Autodesk Fusion 360 part; units mm, degrees
(part 2 of 3)
  arc A65 (20.2, 68) -> (20, 67.8) centre (20.2, 67.8) ccw
  line L946 (26, 62.4) -> (26.5, 62.4)
  line L947 (20, 62.2) -> (20, 63.55)
  line L948 (26, 63.1) -> (26, 62.4)
  arc A66 (37.0205, 29.8133) -> (36.6712, 29.464) centre (37.0205, 29.464) ccw
  line L949 (37.2921, 29.6968) -> (38.0682, 29.0371)
  line L950 (25.75, 68) -> (25.8, 68)
  arc A67 (37.2921, 26.9628) -> (36.6713, 26.9628) centre (36.9817, 26.9628) ccw
  line L951 (37.7578, 23.9571) -> (37.7578, 24.7333)
  line L952 (44.4112, 30.9247) -> (43.7903, 30.9247)
  line L953 (38.0682, 31.3231) -> (38.0682, 32.0993)
  line L954 (44.7993, 33.1153) -> (43.4023, 33.1153)
  line L955 (19.5, 67.6) -> (19.5, 66.9)
  line L956 (36.6713, 31.7112) -> (38.0682, 31.7112)
  arc A68 (43.7903, 31.7008) -> (43.7903, 30.9246) centre (43.7903, 31.3127) ccw
  arc A69 (38.0683, 26.8852) -> (37.2921, 26.8852) centre (37.6802, 26.8852) ccw
  line L957 (38.0682, 26.4971) -> (38.0682, 26.8852)
  arc A70 (26, 67.8) -> (25.8, 68) centre (25.8, 67.8) ccw
  line L958 (44.7993, 32.3391) -> (43.4023, 32.3391)
  line L959 (37.2921, 26.9628) -> (37.2921, 26.6524)
  line L960 (36.6713, 24.2676) -> (37.7578, 23.9571)
  line L961 (38.0682, 29.0371) -> (38.0682, 29.8133)
  arc A71 (36.6712, 29.464) -> (36.9817, 29.0371) centre (37.1199, 29.464) ccw
  line L962 (37.4474, 24.5004) -> (38.0682, 24.5004)
  line L963 (43.4023, 32.3391) -> (44.7993, 33.1153)
  line L964 (20, 63.1) -> (19.5, 63.1)
  line L965 (19.5, 66.9) -> (20, 66.9)
  line L966 (36.6713, 26.4971) -> (36.6713, 26.9628)
  line L967 (26.5, 63.1) -> (26, 63.1)
  line L968 (25.8, 62) -> (25.4, 62)
  line L969 (40.8, 53.3) -> (39.2, 53.3)
  line L970 (36.7, 15.6) -> (38.3, 15.6)
  arc A72 (44.4112, 30.9246) -> (44.4112, 31.7008) centre (44.4112, 31.3127) ccw
  line L971 (39.2, 12) -> (40.8, 12)
  line L972 (43.3, 53.3) -> (41.7, 53.3)
  line L973 (39.2, 15.6) -> (40.8, 15.6)
  line L974 (41.7, 15.6) -> (43.3, 15.6)
  line L975 (38.3, 53.3) -> (36.7, 53.3)
  line L976 (36.9817, 31.3231) -> (36.6713, 31.7112)
  line L977 (41.7, 12) -> (43.3, 12)
  arc A73 (37.2921, 29.6968) -> (37.0205, 29.8132) centre (37.0205, 29.4381) ccw
  line L978 (43.7903, 31.7008) -> (44.4112, 31.7008)
  line L979 (43.3, 49.7) -> (41.7, 49.7)
  line L980 (36.7, 12) -> (38.3, 12)
  line L981 (38.3, 49.7) -> (36.7, 49.7)
  line L982 (40.8, 49.7) -> (39.2, 49.7)
  line L983 (14.5813, 71.8525) -> (14.5813, 70.8525)
  circle A74 centre (15.0813, 71.8525) radius 0.5
  line L984 (15.5813, 70.8525) -> (15.5813, 71.8525)
  line L985 (14.5813, 57.0525) -> (15.5813, 57.0525)
  line L986 (14.5813, 70.8525) -> (15.5813, 70.8525)
  line L987 (15.5813, 71.8525) -> (14.5813, 71.8525)
  line L988 (15.5813, 57.0525) -> (15.5813, 58.0525)
  circle A75 centre (15.0813, 57.0525) radius 0.5
  line L989 (24.714, 14.816) -> (24.714, 15.324)
  line L990 (33.401, 50.419) -> (33.401, 49.911)
  line L991 (24.206, 15.324) -> (24.206, 14.816)
  line L992 (26.746, 14.816) -> (27.254, 14.816)
  line L993 (33.401, 52.959) -> (33.401, 52.451)
  line L994 (33.909, 52.959) -> (33.401, 52.959)
  line L995 (24.714, 15.324) -> (24.206, 15.324)
  line L996 (27.254, 15.324) -> (26.746, 15.324)
  line L997 (14.5813, 58.0525) -> (14.5813, 57.0525)
  line L998 (15.5813, 58.0525) -> (14.5813, 58.0525)
  line L999 (33.909, 50.419) -> (33.401, 50.419)
  line L1000 (33.909, 52.451) -> (33.909, 52.959)
  line L1001 (33.909, 49.911) -> (33.909, 50.419)
  line L1002 (33.401, 49.911) -> (33.909, 49.911)
  line L1003 (33.401, 52.451) -> (33.909, 52.451)
  line L1004 (24.206, 14.816) -> (24.714, 14.816)
  line L1005 (27.254, 14.816) -> (27.254, 15.324)
  line L1006 (24.714, 12.276) -> (24.714, 12.784)
  line L1007 (24.714, 12.784) -> (24.206, 12.784)
  line L1008 (24.206, 12.784) -> (24.206, 12.276)
  line L1009 (24.206, 12.276) -> (24.714, 12.276)
sketch "PET_Diag_Clip" plane through (0, 0, 0) normal (0, 0, 1) x (1, 0, 0) in component "PCB"
  line L0 (0, 0) -> (47, 0)
  line L1 (0, 77) -> (0, 0)
  line L2 (47, 0) -> (47, 77)
  line L3 (47, 77) -> (0, 77)
  line L4 (7.366, 50.434) -> (7.366, 49.926)
  line L5 (7.874, 50.434) -> (7.366, 50.434)
  line L6 (7.874, 47.386) -> (7.874, 47.894)
  line L7 (4.826, 44.846) -> (5.334, 44.846)
  line L8 (7.874, 57.546) -> (7.874, 58.054)
  line L9 (4.826, 55.514) -> (4.826, 55.006)
  line L10 (7.366, 57.546) -> (7.874, 57.546)
  line L11 (4.826, 45.354) -> (4.826, 44.846)
  line L12 (7.874, 58.054) -> (7.366, 58.054)
  line L13 (7.366, 47.894) -> (7.366, 47.386)
  line L14 (4.826, 50.434) -> (4.826, 49.926)
  line L15 (7.366, 52.466) -> (7.874, 52.466)
  line L16 (7.874, 45.354) -> (7.366, 45.354)
  line L17 (7.874, 44.846) -> (7.874, 45.354)
  line L18 (7.874, 55.006) -> (7.874, 55.514)
  line L19 (7.366, 52.974) -> (7.366, 52.466)
  line L20 (5.334, 47.894) -> (4.826, 47.894)
  line L21 (7.366, 49.926) -> (7.874, 49.926)
  line L22 (5.334, 57.546) -> (5.334, 58.054)
  line L23 (5.334, 58.054) -> (4.826, 58.054)
  line L24 (7.874, 42.306) -> (7.874, 42.814)
  line L25 (5.334, 49.926) -> (5.334, 50.434)
  line L26 (7.366, 42.306) -> (7.874, 42.306)
  line L27 (7.366, 58.054) -> (7.366, 57.546)
  line L28 (4.826, 52.466) -> (5.334, 52.466)
  line L29 (7.366, 44.846) -> (7.874, 44.846)
  line L30 (4.826, 57.546) -> (5.334, 57.546)
  line L31 (5.334, 52.466) -> (5.334, 52.974)
  line L32 (5.334, 50.434) -> (4.826, 50.434)
  line L33 (7.874, 60.086) -> (7.874, 60.594)
  line L34 (5.334, 47.386) -> (5.334, 47.894)
  line L35 (5.334, 45.354) -> (4.826, 45.354)
  line L36 (5.334, 55.006) -> (5.334, 55.514)
  line L37 (4.826, 47.894) -> (4.826, 47.386)
  line L38 (7.366, 47.386) -> (7.874, 47.386)
  line L39 (7.366, 55.006) -> (7.874, 55.006)
  line L40 (7.874, 60.594) -> (7.366, 60.594)
  line L41 (4.826, 47.386) -> (5.334, 47.386)
  line L42 (4.826, 55.006) -> (5.334, 55.006)
  line L43 (7.366, 55.514) -> (7.366, 55.006)
  line L44 (4.826, 52.974) -> (4.826, 52.466)
  line L45 (7.874, 52.466) -> (7.874, 52.974)
  line L46 (7.874, 49.926) -> (7.874, 50.434)
  line L47 (5.334, 44.846) -> (5.334, 45.354)
  line L48 (7.366, 42.814) -> (7.366, 42.306)
  line L49 (4.826, 58.054) -> (4.826, 57.546)
  line L50 (5.334, 55.514) -> (4.826, 55.514)
  line L51 (7.874, 52.974) -> (7.366, 52.974)
  line L52 (5.334, 52.974) -> (4.826, 52.974)
  line L53 (7.874, 47.894) -> (7.366, 47.894)
  line L54 (7.874, 55.514) -> (7.366, 55.514)
  line L55 (4.826, 49.926) -> (5.334, 49.926)
  line L56 (4.826, 60.594) -> (4.826, 60.086)
  line L57 (7.366, 45.354) -> (7.366, 44.846)
  line L58 (4.826, 32.654) -> (4.826, 32.146)
  line L59 (7.874, 34.686) -> (7.874, 35.194)
  line L60 (7.366, 34.686) -> (7.874, 34.686)
  line L61 (5.334, 42.814) -> (4.826, 42.814)
  line L62 (4.826, 37.734) -> (4.826, 37.226)
  line L63 (7.366, 39.766) -> (7.874, 39.766)
  line L64 (4.826, 30.114) -> (4.826, 29.606)
  line L65 (7.366, 62.626) -> (7.874, 62.626)
  line L66 (7.366, 60.086) -> (7.874, 60.086)
  line L67 (7.874, 39.766) -> (7.874, 40.274)
  line L68 (7.874, 37.226) -> (7.874, 37.734)
  line L69 (7.874, 40.274) -> (7.366, 40.274)
  line L70 (7.366, 37.734) -> (7.366, 37.226)
  line L71 (7.366, 27.066) -> (7.874, 27.066)
  line L72 (7.874, 37.734) -> (7.366, 37.734)
  line L73 (4.826, 35.194) -> (4.826, 34.686)
  line L74 (5.334, 63.134) -> (4.826, 63.134)
  line L75 (5.334, 35.194) -> (4.826, 35.194)
  line L76 (5.334, 60.086) -> (5.334, 60.594)
  line L77 (5.334, 60.594) -> (4.826, 60.594)
  line L78 (7.874, 27.066) -> (7.874, 27.574)
  line L79 (4.826, 29.606) -> (5.334, 29.606)
  line L80 (4.826, 63.134) -> (4.826, 62.626)
  line L81 (7.874, 27.574) -> (7.366, 27.574)
  line L82 (5.334, 32.654) -> (4.826, 32.654)
  line L83 (4.826, 39.766) -> (5.334, 39.766)
  line L84 (7.366, 30.114) -> (7.366, 29.606)
  line L85 (4.826, 27.574) -> (4.826, 27.066)
  line L86 (7.874, 63.134) -> (7.366, 63.134)
  line L87 (7.366, 60.594) -> (7.366, 60.086)
  line L88 (4.826, 62.626) -> (5.334, 62.626)
  line L89 (5.334, 62.626) -> (5.334, 63.134)
  line L90 (5.334, 34.686) -> (5.334, 35.194)
  line L91 (5.334, 32.146) -> (5.334, 32.654)
  line L92 (4.826, 27.066) -> (5.334, 27.066)
  line L93 (7.366, 29.606) -> (7.874, 29.606)
  line L94 (4.826, 60.086) -> (5.334, 60.086)
  line L95 (7.366, 32.146) -> (7.874, 32.146)
  line L96 (7.366, 63.134) -> (7.366, 62.626)
  line L97 (4.826, 34.686) -> (5.334, 34.686)
  line L98 (7.874, 42.814) -> (7.366, 42.814)
  line L99 (7.366, 35.194) -> (7.366, 34.686)
  line L100 (7.366, 40.274) -> (7.366, 39.766)
  line L101 (7.366, 37.226) -> (7.874, 37.226)
  line L102 (7.874, 62.626) -> (7.874, 63.134)
  line L103 (7.874, 35.194) -> (7.366, 35.194)
  line L104 (5.334, 39.766) -> (5.334, 40.274)
  line L105 (7.874, 30.114) -> (7.366, 30.114)
  line L106 (5.334, 19.954) -> (4.826, 19.954)
  line L107 (7.366, 19.446) -> (7.874, 19.446)
  line L108 (7.366, 14.874) -> (7.366, 14.366)
  line L109 (4.826, 40.274) -> (4.826, 39.766)
  line L110 (4.826, 32.146) -> (5.334, 32.146)
  line L111 (4.826, 25.034) -> (4.826, 24.526)
  line L112 (7.874, 24.526) -> (7.874, 25.034)
  line L113 (4.826, 24.526) -> (5.334, 24.526)
  line L114 (7.366, 27.574) -> (7.366, 27.066)
  line L115 (5.334, 29.606) -> (5.334, 30.114)
  line L116 (4.826, 42.306) -> (5.334, 42.306)
  line L117 (7.366, 25.034) -> (7.366, 24.526)
  line L118 (5.334, 40.274) -> (4.826, 40.274)
  line L119 (5.334, 37.226) -> (5.334, 37.734)
  line L120 (7.366, 14.366) -> (7.874, 14.366)
  line L121 (7.874, 29.606) -> (7.874, 30.114)
  line L122 (7.366, 21.986) -> (7.874, 21.986)
  line L123 (5.334, 37.734) -> (4.826, 37.734)
  line L124 (7.366, 32.654) -> (7.366, 32.146)
  line L125 (4.826, 42.814) -> (4.826, 42.306)
  line L126 (7.874, 16.906) -> (7.874, 17.414)
  line L127 (7.366, 17.414) -> (7.366, 16.906)
  line L128 (5.334, 22.494) -> (4.826, 22.494)
  line L129 (5.334, 30.114) -> (4.826, 30.114)
  line L130 (5.334, 14.874) -> (4.826, 14.874)
  line L131 (7.874, 22.494) -> (7.366, 22.494)
  line L132 (4.826, 37.226) -> (5.334, 37.226)
  line L133 (4.826, 22.494) -> (4.826, 21.986)
  line L134 (7.874, 32.654) -> (7.366, 32.654)
  line L135 (7.874, 32.146) -> (7.874, 32.654)
  line L136 (5.334, 42.306) -> (5.334, 42.814)
  line L137 (7.366, 24.526) -> (7.874, 24.526)
  line L138 (5.334, 24.526) -> (5.334, 25.034)
  line L139 (5.334, 27.066) -> (5.334, 27.574)
  line L140 (5.334, 17.414) -> (4.826, 17.414)
  line L141 (7.366, 16.906) -> (7.874, 16.906)
  line L142 (7.874, 25.034) -> (7.366, 25.034)
  line L143 (4.826, 17.414) -> (4.826, 16.906)
  line L144 (5.334, 14.366) -> (5.334, 14.874)
  line L145 (5.334, 21.986) -> (5.334, 22.494)
  line L146 (5.334, 27.574) -> (4.826, 27.574)
  line L147 (7.874, 14.366) -> (7.874, 14.874)
  line L148 (4.826, 21.986) -> (5.334, 21.986)
  line L149 (7.874, 19.954) -> (7.366, 19.954)
  line L150 (5.334, 19.446) -> (5.334, 19.954)
  line L151 (7.874, 21.986) -> (7.874, 22.494)
  line L152 (7.874, 14.874) -> (7.366, 14.874)
  line L153 (7.366, 22.494) -> (7.366, 21.986)
  line L154 (4.826, 14.874) -> (4.826, 14.366)
  line L155 (5.334, 25.034) -> (4.826, 25.034)
  line L156 (4.826, 16.906) -> (5.334, 16.906)
  line L157 (7.874, 17.414) -> (7.366, 17.414)
  line L158 (4.826, 19.446) -> (5.334, 19.446)
  line L159 (5.334, 16.906) -> (5.334, 17.414)
  line L160 (4.826, 14.366) -> (5.334, 14.366)
  line L161 (7.874, 19.446) -> (7.874, 19.954)
  line L162 (7.366, 19.954) -> (7.366, 19.446)
  line L163 (4.826, 19.954) -> (4.826, 19.446)
  line L164 (17.8813, 69.2525) -> (17.8813, 59.6525)
  line L165 (17.8813, 59.6525) -> (12.2813, 59.6525)
  line L166 (12.2813, 59.6525) -> (12.2813, 69.2525)
  line L167 (12.2813, 69.2525) -> (17.8813, 69.2525)
  circle A0 centre (5, 5) radius 3.1789
  circle A1 centre (5, 5) radius 1.7463
  circle A2 centre (42, 5) radius 3.1789
  circle A3 centre (42, 5) radius 1.7463
  circle A4 centre (42, 72) radius 3.1789
  circle A5 centre (42, 72) radius 1.7463
  circle A6 centre (5, 72) radius 3.1789
  circle A7 centre (5, 72) radius 1.7463
  line L168 (23.3362, 18.542) -> (28.6703, 18.542)
  arc A8 (23.3363, 18.542) -> (20.7963, 18.542) centre (22.0663, 18.542) ccw
  line L169 (28.6703, 53.848) -> (15.4623, 53.848)
  line L170 (15.4623, 18.542) -> (20.7963, 18.542)
  line L171 (15.4623, 18.542) -> (15.4623, 53.848)
  line L172 (28.6703, 18.542) -> (28.6703, 53.848)
  line L173 (35.687, 9.398) -> (16.383, 9.398)
  line L174 (16.383, 3.302) -> (35.687, 3.302)
  line L175 (35.687, 9.398) -> (35.687, 3.302)
  line L176 (16.383, 9.398) -> (16.383, 7.366)
  line L177 (16.383, 3.302) -> (16.383, 5.334)
  arc A9 (16.383, 5.334) -> (16.383, 7.366) centre (16.383, 6.35) ccw
  line L178 (10.9538, 67.96) -> (10.9538, 9.54)
  line L179 (10.9538, 9.54) -> (9.525, 9.54)
  line L180 (9.525, 9.54) -> (8.0963, 9.54)
  line L181 (8.0963, 9.54) -> (1.7462, 9.54)
  line L182 (1.7462, 9.54) -> (1.7462, 36.6862)
  line L183 (1.7462, 36.6862) -> (1.7462, 40.8138)
  line L184 (1.7462, 40.8138) -> (1.7462, 62.0863)
  line L185 (1.7462, 62.0863) -> (1.7462, 62.4038)
  line L186 (1.7462, 62.4038) -> (1.7462, 62.5625)
  line L187 (1.7462, 62.5625) -> (1.7462, 62.7213)
  line L188 (1.7462, 62.7213) -> (1.7462, 62.88)
  line L189 (1.7462, 62.88) -> (1.7462, 63.0388)
  line L190 (1.7462, 63.1975) -> (1.7462, 63.3563)
  line L191 (1.7462, 63.3563) -> (1.7462, 63.515)
  line L192 (1.7462, 63.515) -> (1.7462, 63.6738)
  line L193 (1.7462, 63.6738) -> (1.7462, 67.96)
  line L194 (1.7462, 67.96) -> (8.0963, 67.96)
  line L195 (8.0963, 67.96) -> (9.525, 67.96)
  line L196 (9.525, 67.96) -> (10.9538, 67.96)
  line L197 (9.6838, 66.69) -> (9.6838, 10.81)
  line L198 (9.6838, 10.81) -> (9.525, 10.81)
  line L199 (9.525, 10.81) -> (8.0963, 10.81)
  line L200 (8.0963, 10.81) -> (3.0162, 10.81)
  line L201 (3.0162, 10.81) -> (3.0162, 36.6862)
  line L202 (3.0162, 36.6862) -> (3.0162, 40.8138)
  line L203 (3.0162, 40.8138) -> (3.0162, 66.69)
  line L204 (3.0162, 66.69) -> (8.0963, 66.69)
  line L205 (8.0963, 66.69) -> (9.525, 66.69)
  line L206 (9.525, 66.69) -> (9.6838, 66.69)
  line L207 (3.0162, 40.8138) -> (2.54, 40.8138)
  line L208 (2.54, 40.8138) -> (1.7462, 40.8138)
  line L209 (3.0162, 36.6862) -> (2.54, 36.6862)
  line L210 (2.54, 36.6862) -> (1.7462, 36.6862)
  line L211 (9.525, 10.81) -> (9.525, 10.3337)
  line L212 (9.525, 10.3337) -> (9.525, 9.54)
  line L213 (9.525, 66.69) -> (9.525, 67.1663)
  line L214 (9.525, 67.1663) -> (9.525, 67.96)
  line L215 (8.0963, 66.69) -> (8.0963, 67.1663)
  line L216 (8.0963, 67.1663) -> (8.0963, 67.96)
  line L217 (8.0963, 10.81) -> (8.0963, 10.3337)
  line L218 (8.0963, 10.3337) -> (8.0963, 9.54)
  line L219 (10.16, 67.1663) -> (10.16, 10.3337)
  line L220 (2.54, 36.6862) -> (2.54, 10.3337)
  line L221 (8.0963, 10.3337) -> (2.54, 10.3337)
  line L222 (10.16, 67.1663) -> (9.525, 67.1663)
  line L223 (8.0963, 67.1663) -> (2.54, 67.1663)
  line L224 (2.54, 40.8138) -> (2.54, 62.88)
  line L225 (2.54, 62.88) -> (2.54, 67.1663)
  line L226 (9.525, 10.3337) -> (10.16, 10.3337)
  line L227 (3.0162, 10.81) -> (2.54, 10.3337)
  line L228 (9.6838, 10.81) -> (10.16, 10.3337)
  line L229 (10.16, 67.1663) -> (9.6838, 66.69)
  line L230 (2.54, 67.1663) -> (3.0162, 66.69)
  arc A10 (10.9538, 65.42) -> (10.9538, 66.69) centre (10.9538, 66.055) ccw
  arc A11 (10.9538, 10.81) -> (10.9538, 12.08) centre (10.9538, 11.445) ccw
  arc A12 (10.9538, 38.2738) -> (10.9538, 39.385) centre (10.9538, 38.8294) ccw
  line L231 (2.54, 62.88) -> (1.7462, 63.6738)
  line L232 (2.54, 62.88) -> (2.5399, 62.88)
  line L233 (2.5399, 62.88) -> (2.3812, 62.7213)
  line L234 (2.3812, 62.7213) -> (2.0637, 62.4038)
  line L235 (2.0637, 62.4038) -> (1.7462, 62.0863)
  line L236 (2.3812, 62.88) -> (1.7462, 63.515)
  line L237 (1.7462, 63.3563) -> (2.3812, 62.7213)
  line L238 (2.2225, 62.7213) -> (2.2224, 62.7213)
  line L239 (2.2224, 62.7213) -> (1.7462, 63.1975)
  line L240 (1.7462, 63.1975) -> (1.7462, 63.0388)
  line L241 (1.7462, 63.0388) -> (2.2225, 62.5625)
  line L242 (1.7462, 62.88) -> (2.0637, 62.5625)
  line L243 (1.7462, 62.7213) -> (2.0637, 62.4038)
  line L244 (1.7462, 62.5625) -> (1.7463, 62.5625)
  line L245 (1.7463, 62.5625) -> (1.905, 62.4038)
  line L246 (1.7462, 62.4038) -> (1.905, 62.245)
  arc A13 (38.5, 55.7) -> (41.5, 55.7) centre (40, 56.5) ccw
  arc A14 (41.5, 57.3) -> (38.5, 57.3) centre (40, 56.5) ccw
  arc A15 (38.5, 55.7) -> (41.5, 55.7) centre (40, 56.5) ccw
  arc A16 (41.5, 57.3) -> (38.5, 57.3) centre (40, 56.5) ccw
  line L247 (20.25, 68) -> (25.75, 68)
  line L248 (26, 66.45) -> (26, 63.6)
  line L249 (25.4, 62) -> (20.25, 62)
  line L250 (20, 63.55) -> (20, 66.45)
  arc A17 (20.55, 62.45) -> (20.5, 63.2) centre (20.8502, 62.8467) ccw
  arc A18 (20.55, 66.75) -> (20.5, 67.5) centre (20.8502, 67.1467) ccw
  arc A19 (25.45, 67.55) -> (25.5, 66.8) centre (25.1498, 67.1533) ccw
  arc A20 (25.45, 63.25) -> (25.45, 62.45) centre (25.15, 62.85) ccw
  circle A21 centre (23, 65) radius 1.75
  circle A22 centre (23, 65) radius 1.4
  line L251 (35.8458, 33.9408) -> (35.8458, 22.2568)
  line L252 (45.7518, 22.2568) -> (45.7518, 33.9408)
  line L253 (45.7518, 33.9408) -> (42.4498, 33.9408)
  line L254 (39.1478, 33.9408) -> (39.1478, 33.4327)
  line L255 (39.1478, 33.4327) -> (42.4498, 33.4327)
  line L256 (42.4498, 33.4327) -> (42.4498, 33.9408)
  line L257 (39.1478, 33.9408) -> (35.8458, 33.9408)
  line L258 (42.4498, 33.9408) -> (39.1478, 33.9408)
  line L259 (35.8458, 22.2568) -> (39.1478, 22.2568)
  line L260 (42.4498, 22.2568) -> (42.4498, 22.7647)
  line L261 (42.4498, 22.7647) -> (39.1478, 22.7647)
  line L262 (39.1478, 22.7647) -> (39.1478, 22.2568)
  line L263 (42.4498, 22.2568) -> (45.7518, 22.2568)
  line L264 (39.1478, 22.2568) -> (42.4498, 22.2568)
  line L265 (42.7037, 25.0508) -> (38.8938, 25.0508)
  line L266 (42.7037, 25.0508) -> (42.7037, 23.5267)
  line L267 (38.8938, 23.5267) -> (42.7037, 23.5267)
  line L268 (38.8938, 23.5267) -> (38.8938, 25.0508)
  line L269 (40.7988, 24.7968) -> (39.1478, 24.7968)
  line L270 (40.7988, 23.7808) -> (39.1478, 23.7808)
  line L271 (42.7037, 27.5907) -> (38.8938, 27.5907)
  line L272 (42.7037, 27.5907) -> (42.7037, 26.0668)
  line L273 (38.8938, 26.0668) -> (42.7037, 26.0668)
  line L274 (38.8938, 26.0668) -> (38.8938, 27.5907)
  line L275 (40.7988, 27.3368) -> (39.1478, 27.3368)
  line L276 (40.7988, 26.3208) -> (39.1478, 26.3208)
  line L277 (42.7037, 30.1308) -> (38.8938, 30.1308)
  line L278 (42.7037, 30.1308) -> (42.7037, 28.6068)
  line L279 (38.8938, 28.6068) -> (42.7037, 28.6068)
  line L280 (38.8938, 28.6068) -> (38.8938, 30.1308)
  line L281 (40.7988, 29.8768) -> (39.1478, 29.8768)
  line L282 (40.7988, 28.8608) -> (39.1478, 28.8608)
  line L283 (42.7037, 32.6707) -> (38.8938, 32.6707)
  line L284 (42.7037, 32.6707) -> (42.7037, 31.1468)
  line L285 (38.8938, 31.1468) -> (42.7037, 31.1468)
  line L286 (38.8938, 31.1468) -> (38.8938, 32.6707)
  line L287 (40.7988, 32.4168) -> (39.1478, 32.4168)
  line L288 (40.7988, 31.4008) -> (39.1478, 31.4008)
  line L289 (35.5, 15.6) -> (35.5, 12)
  line L290 (35.5, 12) -> (36.7, 12)
  line L291 (35.5, 15.6) -> (36.7, 15.6)
  line L292 (44.6, 12) -> (44.6, 15.6)
  line L293 (44.6, 15.6) -> (43.3, 15.6)
  line L294 (44.6, 12) -> (43.3, 12)
  line L295 (38.3, 15.6) -> (39.2, 15.6)
  line L296 (40.8, 15.6) -> (41.7, 15.6)
  line L297 (38.3, 12) -> (39.2, 12)
  line L298 (40.8, 12) -> (41.7, 12)
  line L299 (38.3, 14.5) -> (38.3, 13.1)
  line L300 (38.3, 13.1) -> (41.7, 13.1)
  line L301 (41.7, 13.1) -> (41.7, 14.5)
  line L302 (41.7, 14.5) -> (38.3, 14.5)
  line L303 (31.35, 77) -> (23.5, 77)
  line L304 (23.5, 77) -> (15.65, 77)
  line L305 (31.35, 77) -> (31.35, 83.5)
  line L306 (15.65, 77) -> (15.65, 83.5)
  line L307 (35.15, 83.9) -> (23.85, 83.9)
  line L308 (23.85, 83.9) -> (18.85, 83.9)
  line L309 (18.85, 83.9) -> (11.85, 83.9)
  line L310 (35.15, 83.5) -> (11.85, 83.5)
  line L311 (11.85, 83.9) -> (11.85, 83.5)
  line L312 (35.15, 83.9) -> (35.15, 83.5)
  line L313 (18.85, 83.9) -> (18.85, 88.4)
  line L314 (21.35, 88.9) -> (20.85, 88.4)
  line L315 (20.85, 88.4) -> (20.35, 88.9)
  line L316 (20.35, 88.9) -> (19.85, 88.4)
  line L317 (19.85, 88.4) -> (19.35, 88.9)
  line L318 (21.35, 88.9) -> (21.85, 88.4)
  line L319 (21.85, 88.4) -> (22.35, 88.9)
  line L320 (22.35, 88.9) -> (22.85, 88.4)
  line L321 (22.85, 88.4) -> (23.35, 88.9)
  line L322 (19.35, 88.9) -> (18.85, 88.4)
  line L323 (23.35, 88.9) -> (23.85, 88.4)
  line L324 (23.85, 88.4) -> (23.85, 83.9)
  line L325 (33, 86) -> (33, 84.5)
  line L326 (33, 83.5) -> (33, 82)
  line L327 (14, 86) -> (14, 84.5)
  line L328 (14, 83.5) -> (14, 82)
  line L329 (12.2813, 61.4525) -> (12.2813, 60.4525)
  line L330 (17.8813, 60.4525) -> (17.8813, 61.4525)
  line L331 (17.8813, 61.4525) -> (12.2813, 61.4525)
  line L332 (12.2813, 60.4525) -> (17.8813, 60.4525)
  line L333 (15.5813, 58.0525) -> (15.5813, 59.6525)
  line L334 (15.5813, 70.8525) -> (14.5813, 70.8525)
  line L335 (14.5813, 58.0525) -> (15.5813, 58.0525)
  line L336 (15.5813, 59.6525) -> (14.5813, 59.6525)
  line L337 (14.5813, 59.6525) -> (14.5813, 58.0525)
  line L338 (14.5813, 69.2525) -> (15.5813, 69.2525)
  line L339 (15.5813, 69.2525) -> (15.5813, 70.8525)
  line L340 (14.5813, 70.8525) -> (14.5813, 69.2525)
  line L341 (40.1638, 29.8768) -> (39.7828, 29.8768)
  line L342 (40.4178, 26.3208) -> (40.7988, 26.3208)
  line L343 (40.1638, 27.3368) -> (39.7828, 27.3368)
  line L344 (39.1478, 24.7968) -> (39.1478, 23.7808)
  line L345 (40.1638, 31.4008) -> (40.1638, 32.4168)
  line L346 (39.1478, 32.4168) -> (39.1478, 31.4008)
  line L347 (39.7828, 29.8768) -> (39.7828, 28.8608)
  line L348 (39.7828, 24.7968) -> (39.7828, 23.7808)
  line L349 (39.5288, 24.7968) -> (39.1478, 24.7968)
  line L350 (40.4178, 28.8608) -> (40.7988, 28.8608)
  line L351 (40.4178, 31.4008) -> (40.7988, 31.4008)
  line L352 (40.7988, 26.3208) -> (40.7988, 27.3368)
  line L353 (40.1638, 24.7968) -> (39.7828, 24.7968)
  line L354 (40.4178, 27.3368) -> (40.4178, 26.3208)
  line L355 (40.1638, 23.7808) -> (40.1638, 24.7968)
  line L356 (39.7828, 27.3368) -> (39.7828, 26.3208)
  line L357 (39.5288, 26.3208) -> (39.5288, 27.3368)
  line L358 (39.1478, 26.3208) -> (39.5288, 26.3208)
  line L359 (40.7988, 27.3368) -> (40.4178, 27.3368)
  line L360 (40.1638, 26.3208) -> (40.1638, 27.3368)
  line L361 (40.7988, 24.7968) -> (40.4178, 24.7968)
  line L362 (40.7988, 28.8608) -> (40.7988, 29.8768)
  line L363 (39.7828, 26.3208) -> (40.1638, 26.3208)
  line L364 (40.7988, 29.8768) -> (40.4178, 29.8768)
  line L365 (39.1478, 23.7808) -> (39.5288, 23.7808)
  line L366 (39.5288, 27.3368) -> (39.1478, 27.3368)
  line L367 (40.4178, 24.7968) -> (40.4178, 23.7808)
  line L368 (40.1638, 28.8608) -> (40.1638, 29.8768)
  line L369 (39.1478, 28.8608) -> (39.5288, 28.8608)
  line L370 (39.1478, 27.3368) -> (39.1478, 26.3208)
  line L371 (39.7828, 31.4008) -> (40.1638, 31.4008)
  line L372 (39.5288, 28.8608) -> (39.5288, 29.8768)
  line L373 (39.5288, 32.4168) -> (39.1478, 32.4168)
  line L374 (39.7828, 28.8608) -> (40.1638, 28.8608)
  line L375 (40.4178, 29.8768) -> (40.4178, 28.8608)
  line L376 (40.7988, 32.4168) -> (40.4178, 32.4168)
  line L377 (39.1478, 31.4008) -> (39.5288, 31.4008)
  line L378 (39.5288, 31.4008) -> (39.5288, 32.4168)
  line L379 (39.1478, 29.8768) -> (39.1478, 28.8608)
  line L380 (39.5288, 29.8768) -> (39.1478, 29.8768)
  line L381 (40.7988, 31.4008) -> (40.7988, 32.4168)
  line L382 (40.1638, 32.4168) -> (39.7828, 32.4168)
  line L383 (40.7988, 23.7808) -> (40.7988, 24.7968)
  line L384 (39.5288, 23.7808) -> (39.5288, 24.7968)
  line L385 (39.7828, 23.7808) -> (40.1638, 23.7808)
  line L386 (40.4178, 32.4168) -> (40.4178, 31.4008)
  line L387 (39.7828, 32.4168) -> (39.7828, 31.4008)
  line L388 (40.4178, 23.7808) -> (40.7988, 23.7808)
  line L389 (40.3, 14.5) -> (40.3, 13.1)
  line L390 (41.7, 14.5) -> (40.3, 14.5)
  line L391 (40.3, 13.1) -> (41.7, 13.1)
  line L392 (41.7, 13.1) -> (41.7, 14.5)
  line L393 (19.5, 67.6) -> (19.5, 66.9)
  line L394 (15.5813, 57.0525) -> (15.5813, 58.0525)
  line L395 (15.5813, 58.0525) -> (14.5813, 58.0525)
  line L396 (26, 66.9) -> (26.5, 66.9)
  line L397 (26, 62.4) -> (26.5, 62.4)
  line L398 (26.5, 62.4) -> (26.5, 63.1)
  line L399 (15.5813, 70.8525) -> (15.5813, 71.8525)
  line L400 (14.5813, 58.0525) -> (14.5813, 57.0525)
  line L401 (14.5813, 57.0525) -> (15.5813, 57.0525)
  line L402 (14.5813, 70.8525) -> (15.5813, 70.8525)
  line L403 (26.5, 63.1) -> (26, 63.1)
  line L404 (20, 63.1) -> (19.5, 63.1)
  line L405 (26, 63.1) -> (26, 62.4)
  line L406 (20, 66.9) -> (20, 67.6)
  line L407 (20, 67.6) -> (19.5, 67.6)
  line L408 (19.5, 66.9) -> (20, 66.9)
  line L409 (19.5, 63.1) -> (19.5, 62.4)
  line L410 (26, 67.6) -> (26, 66.9)
  line L411 (20, 62.4) -> (20, 63.1)
  line L412 (26.5, 66.9) -> (26.5, 67.6)
  line L413 (15.5813, 71.8525) -> (14.5813, 71.8525)
  line L414 (19.5, 62.4) -> (20, 62.4)
  line L415 (26.5, 67.6) -> (26, 67.6)
  line L416 (14.5813, 71.8525) -> (14.5813, 70.8525)
  circle A23 centre (15.0813, 57.0525) radius 0.5
  circle A24 centre (15.0813, 71.8525) radius 0.5
  line L417 (38.5, 55.7) -> (38.5, 57.3)
  arc A25 (41.5, 55.7) -> (41.5, 57.3) centre (40, 56.5) ccw
  circle A26 centre (40, 56.5) radius 1.5
  line L418 (20, 66.45) -> (20, 67.8)
  arc A27 (20.2, 68) -> (20, 67.8) centre (20.2, 67.8) ccw
  line L419 (20.2, 68) -> (20.25, 68)
  line L420 (25.75, 68) -> (25.8, 68)
  arc A28 (26, 67.8) -> (25.8, 68) centre (25.8, 67.8) ccw
  line L421 (26, 67.8) -> (26, 66.45)
  line L422 (26, 63.6) -> (26, 62.2)
  arc A29 (25.8, 62) -> (26, 62.2) centre (25.8, 62.2) ccw
  line L423 (25.8, 62) -> (25.4, 62)
  line L424 (20.25, 62) -> (20.2, 62)
  arc A30 (20, 62.2) -> (20.2, 62) centre (20.2, 62.2) ccw
  line L425 (20, 62.2) -> (20, 63.55)
  arc A31 (20.5, 63.2) -> (20.55, 62.45) centre (20.8502, 62.8467) ccw
  arc A32 (20.5, 67.5) -> (20.55, 66.75) centre (20.8502, 67.1467) ccw
  arc A33 (25.5, 66.8) -> (25.45, 67.55) centre (25.1498, 67.1533) ccw
  arc A34 (25.45, 62.45) -> (25.45, 63.25) centre (25.15, 62.85) ccw
  line L426 (36.9817, 31.3231) -> (36.6713, 31.7112)
  line L427 (36.6713, 31.7112) -> (38.0682, 31.7112)
  line L428 (38.0682, 31.3231) -> (38.0682, 32.0993)
  line L429 (44.4112, 30.9247) -> (43.7903, 30.9247)
  arc A35 (43.7903, 31.7008) -> (43.7903, 30.9246) centre (43.7903, 31.3127) ccw
  line L430 (43.7903, 31.7008) -> (44.4112, 31.7008)
  arc A36 (44.4112, 30.9246) -> (44.4112, 31.7008) centre (44.4112, 31.3127) ccw
  line L431 (44.7993, 32.3391) -> (43.4023, 32.3391)
  line L432 (43.4023, 32.3391) -> (44.7993, 33.1153)
  line L433 (44.7993, 33.1153) -> (43.4023, 33.1153)
  arc A37 (37.0205, 29.8133) -> (36.6712, 29.464) centre (37.0205, 29.464) ccw
  arc A38 (36.6712, 29.464) -> (36.9817, 29.0371) centre (37.1199, 29.464) ccw
  arc A39 (37.2921, 29.6968) -> (37.0205, 29.8132) centre (37.0205, 29.4381) ccw
  line L434 (37.2921, 29.6968) -> (38.0682, 29.0371)
  line L435 (38.0682, 29.0371) -> (38.0682, 29.8133)
  line L436 (38.0682, 26.4971) -> (38.0682, 26.8852)
  arc A40 (38.0683, 26.8852) -> (37.2921, 26.8852) centre (37.6802, 26.8852) ccw
  line L437 (36.6713, 26.4971) -> (36.6713, 26.9628)
  arc A41 (37.2921, 26.9628) -> (36.6713, 26.9628) centre (36.9817, 26.9628) ccw
  line L438 (37.2921, 26.9628) -> (37.2921, 26.6524)
  line L439 (36.6713, 24.2676) -> (37.7578, 23.9571)
  line L440 (37.7578, 23.9571) -> (37.7578, 24.7333)
  line L441 (37.4474, 24.5004) -> (38.0682, 24.5004)
  line L442 (44.7993, 23.9663) -> (44.7993, 23.3454)
  line L443 (44.7993, 23.3454) -> (43.4023, 23.3454)
  line L444 (43.4023, 23.3454) -> (43.4023, 23.9663)
  line L445 (44.0231, 23.3454) -> (44.0231, 23.8111)
  line L446 (44.7993, 24.529) -> (43.4023, 24.529)
  line L447 (43.4023, 24.529) -> (43.4023, 24.9171)
  arc A42 (43.7903, 25.3052) -> (43.4022, 24.9171) centre (43.7903, 24.9171) ccw
  line L448 (43.7903, 25.3051) -> (44.4112, 25.3051)
  arc A43 (44.7993, 24.9171) -> (44.4112, 25.3052) centre (44.4112, 24.9171) ccw
  line L449 (44.7993, 24.9171) -> (44.7993, 24.529)
  line L450 (44.0231, 26.5324) -> (44.0231, 26.7653)
  line L451 (44.0231, 26.7653) -> (44.7993, 26.7653)
  line L452 (44.7993, 26.7653) -> (44.7993, 26.2996)
  arc A44 (44.4888, 25.9892) -> (44.7992, 26.2996) centre (44.4888, 26.2996) ccw
  line L453 (44.4888, 25.9891) -> (43.7127, 25.9891)
  arc A45 (43.4022, 26.2996) -> (43.7127, 25.9891) centre (43.7127, 26.2996) ccw
  line L454 (43.4023, 26.2996) -> (43.4023, 26.7653)
  line L455 (36.7, 15.6) -> (38.3, 15.6)
  line L456 (39.2, 15.6) -> (40.8, 15.6)
  line L457 (41.7, 15.6) -> (43.3, 15.6)
  line L458 (36.7, 12) -> (38.3, 12)
  line L459 (39.2, 12) -> (40.8, 12)
  line L460 (41.7, 12) -> (43.3, 12)
  line L461 (24.4, 77) -> (24.4, 73.9)
  line L462 (22.6, 73.9) -> (22.6, 77)
  arc A46 (22.6, 73.9) -> (24.4, 73.9) centre (23.5, 73.9) ccw
  line L463 (24, 75.5) -> (24, 74.5)
  line L464 (23, 74.5) -> (23, 75.5)
  arc A47 (23, 74.5) -> (24, 74.5) centre (23.5, 74.5) ccw
  arc A48 (24, 75.5) -> (23, 75.5) centre (23.5, 75.5) ccw
  line L465 (28.4, 77) -> (28.4, 73.9)
  line L466 (26.6, 73.9) -> (26.6, 77)
  arc A49 (26.6, 73.9) -> (28.4, 73.9) centre (27.5, 73.9) ccw
  line L467 (28, 75.5) -> (28, 74.5)
  line L468 (27, 74.5) -> (27, 75.5)
  arc A50 (27, 74.5) -> (28, 74.5) centre (27.5, 74.5) ccw
  arc A51 (28, 75.5) -> (27, 75.5) centre (27.5, 75.5) ccw
  line L469 (20.5, 77) -> (20.5, 73.9)
  line L470 (18.7, 73.9) -> (18.7, 77)
  arc A52 (18.7, 73.9) -> (20.5, 73.9) centre (19.6, 73.9) ccw
  line L471 (20.1, 75.5) -> (20.1, 74.5)
  line L472 (19.1, 74.5) -> (19.1, 75.5)
  arc A53 (19.1, 74.5) -> (20.1, 74.5) centre (19.6, 74.5) ccw
  arc A54 (20.1, 75.5) -> (19.1, 75.5) centre (19.6, 75.5) ccw
extrude "Extrude1" add sketch "dxf" against normal blind 1.6 contours L0 L1 L2 L3 L450 L451 L452 L453 | L4 L36 L495 L513 L515 L529 L561 | L5 L11 L484 L487 L525 L530 L561 | L17 L19 L509 L513 L529 L542 L582 | L6 L22 L95 L476 L513 L514 L522 L525 L578 | L7 L15 L52 L63 L90 L517 L520 L524 L527 L530 L597 | L31 L90 L95 L109 L113 L518 L522 L535 L539 L597 | L35 L58 L497 L541 L562 L578 L582 | L33 L56 L63 L113 L502 L516 L527 L535 | L22 L32 L37 L40 L85 L109 L473 L501 L508 L514 L518 L526 | L9 L482 L562 L578 | L10 L33 L50 L52 L55 L114 L498 L502 L503 L507 L512 L517 | L29 L30 L31 L38 L41 L42 L44 L56 L85 L114 L499 L501 L507 L516 L519 L523 L536 L539 L543 L575 | L12 L23 L46 L53 L55 L59 L61 L89 L485 L486 L498 L506 L510 L528 L533 L552 | L21 L24 L28 L37 L39 L79 L468 L469 L504 L526 L531 L555 | L25 L40 L42 L79 L505 L508 L543 L555 | L29 L50 L57 L61 L503 L519 L521 L533 | L25 L28 L44 L111 L499 L504 L505 L544 | L23 L41 L57 L86 L510 L521 L532 L575 | A8 L59 L485 A45 | L18 L21 L30 L49 L53 L111 L477 L528 L531 L536 L540 L544 | L38 L46 L49 L86 L523 L532 L540 L552 | A4 L59 L485 A43 | L59 A12 L485 A46 | A0 L16 L20 L45 L47 L51 A34 L464 L467 L475 L490 L493 | A1 L8 L13 L14 L26 L34 L466 L470 L474 L481 L494 A44 | A2 A40 | A3 A38 | L27 L74 L112 L116 L549 L570 L590 L620 | L48 L54 L73 L110 L546 L563 L581 L583 | A10 A36 | A11 A42 | L64 L69 L77 L107 L554 L593 L629 L635 | L65 L83 L94 L123 L556 L579 L586 L596 | L66 L67 L75 L84 L545 L553 L573 L608 | L68 L71 L102 L175 L558 L587 L589 L637 | L70 L78 L96 L118 L548 L551 L569 L588 | L72 L108 L115 L135 L565 L568 L572 L591 | L76 L97 L98 L141 L550 L557 L560 L585 | L80 L99 L101 L104 L564 L592 L595 L612 | L81 L88 L91 L100 L559 L577 L580 L634 | L82 L92 L119 L176 L567 L576 L594 L613 | L87 L105 L106 L122 L598 L615 L621 L622 | L93 L103 L144 L146 L604 L617 L619 L625 | L117 L120 L121 L128 L599 L601 L609 L631 | L124 L147 L150 L178 L606 L623 L651 L657 | L125 L127 L145 L152 L638 L642 L654 L663 | L126 L137 L155 L177 L639 L652 L659 L660 | L129 L162 L165 L183 L602 L611 L636 L646 | L130 L140 L148 L151 L627 L640 L641 L656 | L131 L149 L163 L179 L607 L624 L632 L648 | L132 L167 L170 L180 L610 L633 L653 L655 | L133 L164 L168 L173 L647 L658 L679 L681 | L134 L136 L166 L181 L605 L626 L630 L644 | L138 L161 L169 L182 L600 L603 L643 L661 | L139 L142 L143 L186 L614 L618 L645 L650 | L153 L158 L238 L243 L688 L696 L699 L705 | L154 L157 L171 L198 L667 L680 L698 L700 | L156 L184 L217 L246 L665 L671 L686 L702 | L159 L160 L185 L187 L616 L628 L649 L662 | L172 L188 L195 L225 L668 L685 L689 L697 | L174 L228 L229 L231 L691 L692 L693 L708 | L189 L215 L223 L248 L251 L252 L254 L364 L365 L377 L566 L711 L717 L744 L750 L759 L769 L772 L778 | L191 L222 L224 L250 L262 L269 L270 L365 L374 L378 L731 L736 L740 L742 L751 L759 L764 L776 | L190 L265 L710 L738 | L190 L200 L221 L232 L249 L716 L738 L760 L766 L775 | L205 L259 L261 L726 L738 L753 | L200 L232 L265 L713 L716 L767 | L204 L249 L253 L734 L766 L775 | L193 L255 L259 L264 L265 L710 L726 L739 L741 L753 | L193 L255 L264 L712 L739 L741 L743 L770 | L201 L221 L734 L760 | L192 L221 L263 L730 L745 L771 | L192 L201 L260 L263 L724 L730 L734 L737 L762 | L196 L213 L258 L260 L263 L266 L724 L730 L737 L762 | L194 L208 L216 L218 L676 L678 L684 L709 | L197 L206 L209 L240 L674 L682 L703 L707 | L199 L234 L242 L247 L701 L721 L722 L723 | L202 L203 L219 L237 L664 L672 L675 L719 | L207 L227 L230 L244 L673 L683 L715 L718 | L210 L211 L212 L241 L666 L670 L690 L694 | L214 L226 L233 L245 L669 L704 L706 L720 | L220 L235 L236 L239 L677 L687 L695 L714 | A13 A51 | A14 A20 A55 A63 | L256 L271 L274 L288 L297 L783 L789 L798 L801 L802 L803 L805 L814 L817 L819 L820 L824 | L271 L288 L297 L311 L781 L798 L802 L819 | L783 L788 L801 L803 | L257 L267 L268 L272 L384 L388 L389 L390 L391 L392 A22 A23 L404 L406 L408 L418 L420 A25 L426 A26 L800 L812 L813 L831 L920 A58 L923 L931 L932 L936 L941 L943 L945 A64 A65 L947 L948 L950 A70 L968 | L388 L390 L393 L409 L427 L921 L932 L936 L938 L939 | L387 L389 L396 L397 L420 L931 L944 L946 L948 L967 | L395 L404 L408 L411 L419 L923 L937 L945 L955 L965 | L385 L386 L391 L400 L418 L933 L934 L941 L947 L964 | A15 A21 A56 A57 | A16 A53 | A17 A24 A52 A62 | L273 L275 L279 L286 L289 L301 L307 L410 L442 L447 L787 L807 L822 L826 | L276 L277 L278 L282 L283 L304 L308 L405 L412 L433 L784 L793 L794 L847 | L280 L313 L319 L322 L336 L356 L806 L809 L843 L870 L879 L884 | L280 L313 L322 L327 L806 L809 L852 L884 | L280 L313 L327 L330 L357 L359 L806 L809 L852 L864 L887 L888 | L280 L313 L323 L357 L806 L809 L851 L864 | L280 L313 L320 L323 L332 L350 L806 L809 L834 L836 L851 L886 | L281 L285 L290 L295 L296 L300 L309 L403 L407 L439 L785 L790 L792 L804 | L284 L292 L315 L328 L333 L353 L815 L825 L838 L846 L848 L885 | L284 L292 L333 L349 L815 L825 L863 L885 | L284 L292 L331 L337 L345 L349 L815 L825 L854 L863 L865 L873 | L284 L292 L345 L346 L815 L825 L854 L866 | L284 L292 L294 L346 L348 L360 L815 L825 L853 L856 L866 L882 | L287 L293 L338 L344 L354 L355 L821 L830 L832 L837 L841 L859 | L287 L293 L355 L358 L821 L830 L839 L841 | L287 L293 L314 L326 L329 L358 L821 L830 L835 L839 L858 L883 | L287 L293 L314 L325 L821 L830 L858 L880 | L287 L293 L318 L325 L347 L351 L821 L830 L868 L871 L880 L881 | L291 L298 L299 L303 L306 L310 L312 L401 L413 L438 L791 L795 L823 L829 | A18 A19 A54 A61 | L302 L305 L316 L334 L340 L342 L827 L828 L861 L867 L876 L877 | L302 L305 L340 L341 L827 L828 L844 L861 | L302 L305 L321 L339 L341 L343 L827 L828 L842 L844 L855 L860 | L302 L305 L321 L335 L827 L828 L842 L872 | L302 L305 L317 L324 L335 L352 L827 L828 L833 L845 L869 L872 | L361 L382 L1007 L1008 | L361 L382 L1006 L1007 L1008 L1009 | L361 L362 L366 L382 L1007 L1008 | L363 L367 L371 L379 L993 L994 L1000 L1003 | L368 L428 L991 L995 | L368 L428 L989 L991 L995 L1004 | L368 L399 L421 L428 L991 L995 | L369 L372 L398 L414 L917 L922 | L369 L398 L917 L922 | L369 L398 L917 L922 L925 L942 | L370 L402 L415 L425 L919 L930 | L402 L415 L919 L930 | L402 L415 L919 L928 L929 L930 | L373 L423 L926 L935 | L373 L423 L924 L926 L935 L940 | L373 L394 L417 L423 L926 L935 | L375 L376 L380 L381 L990 L999 L1001 L1002 | L383 L422 L927 L996 | L383 L422 L927 L992 L996 L1005 | L383 L416 L422 L424 L927 L996 | L432 A29 L443 A33 L952 A68 A72 L978 | L454 L455 L458 L460 | L456 L457 L459 L492 | L461 L478 L479 L488 L537 | L461 L478 L489 L491 L496 L986 | L462 L479 L483 L488 L511 L537 | L491 L983 A74 L984 L986 | L463 L472 L479 L488 L511 | A74 L987 | A74 L987 | L463 L465 L471 L472 L480 L998 | L480 L988 A75 L997 L998 | L985 A75 | L985 A75 | A59 | A47 A48 A49 A50 L918 A60 | L725 L780 L796 L818 | L727 L728 L729 L746 L763 L773 | L729 L732 L757 L763 L774 L779 | L728 L746 L786 L810 L816 | L749 L755 L757 L761 L774 L797 | L752 L755 L761 L765 L782 | L840 L850 L874 L891 L897 L903 L906 L907 L910 L916 L969 L972 L975 L979 L981 L982 | L849 L895 L902 L904 L905 L908 L913 | L849 L892 L895 L905 | L857 L875 L878 L899 L900 L901 L909 L911 L912 L914 L970 L971 L973 L974 L977 L980 | L862 L890 L893 L894 L896 L898 L915 | L889 L890 L896 L915 makes body 1 in component "PCB"
extrude "Extrude2" add sketch "dxf" along normal blind 9.5 contours A0 L16 L20 L45 L47 L51 A34 L464 L467 L475 L490 L493 | A1 L8 L13 L14 L26 L34 L466 L470 L474 L481 L494 A44 bodies 1 in component "PCB"
extrude "Extrude3" add sketch "dxf" along normal blind 6 contours L256 L271 L274 L288 L297 L783 L789 L798 L801 L802 L803 L805 L814 L817 L819 L820 L824 | L432 A29 L443 A33 L952 A68 A72 L978 bodies 1 in component "PCB"
extrude "Extrude4" add sketch "dxf" along normal blind 5 contours L273 L275 L279 L286 L289 L301 L307 L410 L442 L447 L787 L807 L822 L826 | L276 L277 L278 L282 L283 L304 L308 L405 L412 L433 L784 L793 L794 L847 | L281 L285 L290 L295 L296 L300 L309 L403 L407 L439 L785 L790 L792 L804 | L291 L298 L299 L303 L306 L310 L312 L401 L413 L438 L791 L795 L823 L829 bodies 1 in component "PCB"
extrude "Extrude5" add sketch "dxf" along normal blind 6.5 contours L280 L313 L319 L322 L336 L356 L806 L809 L843 L870 L879 L884 | L280 L313 L322 L327 L806 L809 L852 L884 | L280 L313 L327 L330 L357 L359 L806 L809 L852 L864 L887 L888 | L280 L313 L323 L357 L806 L809 L851 L864 | L280 L313 L320 L323 L332 L350 L806 L809 L834 L836 L851 L886 | L284 L292 L315 L328 L333 L353 L815 L825 L838 L846 L848 L885 | L284 L292 L333 L349 L815 L825 L863 L885 | L284 L292 L331 L337 L345 L349 L815 L825 L854 L863 L865 L873 | L284 L292 L345 L346 L815 L825 L854 L866 | L284 L292 L294 L346 L348 L360 L815 L825 L853 L856 L866 L882 | L287 L293 L338 L344 L354 L355 L821 L830 L832 L837 L841 L859 | L287 L293 L355 L358 L821 L830 L839 L841 | L287 L293 L314 L326 L329 L358 L821 L830 L835 L839 L858 L883 | L287 L293 L314 L325 L821 L830 L858 L880 | L287 L293 L318 L325 L347 L351 L821 L830 L868 L871 L880 L881 | L302 L305 L316 L334 L340 L342 L827 L828 L861 L867 L876 L877 | L302 L305 L340 L341 L827 L828 L844 L861 | L302 L305 L321 L339 L341 L343 L827 L828 L842 L844 L855 L860 | L302 L305 L321 L335 L827 L828 L842 L872 | L302 L305 L317 L324 L335 L352 L827 L828 L833 L845 L869 L872 bodies 1 in component "PCB"
extrude "Extrude8" add sketch "dxf" along normal blind 9.5 contours L27 L74 L112 L116 L549 L570 L590 L620 | L48 L54 L73 L110 L546 L563 L581 L583 | L64 L69 L77 L107 L554 L593 L629 L635 | L65 L83 L94 L123 L556 L579 L586 L596 | L66 L67 L75 L84 L545 L553 L573 L608 | L68 L71 L102 L175 L558 L587 L589 L637 | L70 L78 L96 L118 L548 L551 L569 L588 | L72 L108 L115 L135 L565 L568 L572 L591 | L76 L97 L98 L141 L550 L557 L560 L585 | L80 L99 L101 L104 L564 L592 L595 L612 | L81 L88 L91 L100 L559 L577 L580 L634 | L82 L92 L119 L176 L567 L576 L594 L613 | L87 L105 L106 L122 L598 L615 L621 L622 | L93 L103 L144 L146 L604 L617 L619 L625 | L117 L120 L121 L128 L599 L601 L609 L631 | L124 L147 L150 L178 L606 L623 L651 L657 | L125 L127 L145 L152 L638 L642 L654 L663 | L126 L137 L155 L177 L639 L652 L659 L660 | L129 L162 L165 L183 L602 L611 L636 L646 | L130 L140 L148 L151 L627 L640 L641 L656 | L131 L149 L163 L179 L607 L624 L632 L648 | L132 L167 L170 L180 L610 L633 L653 L655 | L133 L164 L168 L173 L647 L658 L679 L681 | L134 L136 L166 L181 L605 L626 L630 L644 | L138 L161 L169 L182 L600 L603 L643 L661 | L139 L142 L143 L186 L614 L618 L645 L650 | L153 L158 L238 L243 L688 L696 L699 L705 | L154 L157 L171 L198 L667 L680 L698 L700 | L156 L184 L217 L246 L665 L671 L686 L702 | L159 L160 L185 L187 L616 L628 L649 L662 | L172 L188 L195 L225 L668 L685 L689 L697 | L174 L228 L229 L231 L691 L692 L693 L708 | L194 L208 L216 L218 L676 L678 L684 L709 | L197 L206 L209 L240 L674 L682 L703 L707 | L199 L234 L242 L247 L701 L721 L722 L723 | L202 L203 L219 L237 L664 L672 L675 L719 | L207 L227 L230 L244 L673 L683 L715 L718 | L210 L211 L212 L241 L666 L670 L690 L694 | L214 L226 L233 L245 L669 L704 L706 L720 | L220 L235 L236 L239 L677 L687 L695 L714 bodies 1 in component "PCB"
extrude "Extrude9" add sketch "dxf" along normal blind 2 contours L22 L32 L37 L40 L85 L109 L473 L501 L508 L514 L518 L526 | L10 L33 L50 L52 L55 L114 L498 L502 L503 L507 L512 L517 | L29 L30 L31 L38 L41 L42 L44 L56 L85 L114 L499 L501 L507 L516 L519 L523 L536 L539 L543 L575 | L18 L21 L30 L49 L53 L111 L477 L528 L531 L536 L540 L544 bodies 1 in component "PCB"
extrude "Extrude10" add sketch "dxf" along normal blind 9.5 contours L4 L36 L495 L513 L515 L529 L561 | L5 L11 L484 L487 L525 L530 L561 | L17 L19 L509 L513 L529 L542 L582 | L6 L22 L95 L476 L513 L514 L522 L525 L578 | L7 L15 L52 L63 L90 L517 L520 L524 L527 L530 L597 | L31 L90 L95 L109 L113 L518 L522 L535 L539 L597 | L35 L58 L497 L541 L562 L578 L582 | L33 L56 L63 L113 L502 L516 L527 L535 | L9 L482 L562 L578 | L12 L23 L46 L53 L55 L59 L61 L89 L485 L486 L498 L506 L510 L528 L533 L552 | L21 L24 L28 L37 L39 L79 L468 L469 L504 L526 L531 L555 | L25 L40 L42 L79 L505 L508 L543 L555 | L29 L50 L57 L61 L503 L519 L521 L533 | L25 L28 L44 L111 L499 L504 L505 L544 | L23 L41 L57 L86 L510 L521 L532 L575 | A8 L59 L485 A45 | L38 L46 L49 L86 L523 L532 L540 L552 | A4 L59 L485 A43 | L59 A12 L485 A46 bodies 1 in component "PCB"
extrude "Extrude11" add sketch "dxf" along normal blind 12 contours A59 bodies 1 in component "PCB"
extrude "Extrude12" add sketch "dxf" along normal blind 6.3 contours A47 A48 A49 A50 L918 A60 bodies 1 in component "PCB"
fillet "Fillet2" radius 1.4 1 edges at (38.6015, 55.9576, 12) on bodies 1 in component "PCB"
extrude "Extrude13" add sketch "dxf" along normal blind 12 contours A13 A51 | A16 A53 bodies 1 in component "PCB"
chamfer "Chamfer1" distance 0.25 distance2 9 1 edges at (21.3684, 64.3672, 12) measured on face at (23.482, 65.5025, 12) on bodies 1 in component "PCB"
extrude "Extrude14" add sketch "dxf" along normal blind 4 contours L257 L267 L268 L272 L384 L388 L389 L390 L391 L392 A22 A23 L404 L406 L408 L418 L420 A25 L426 A26 L800 L812 L813 L831 L920 A58 L923 L931 L932 L936 L941 L943 L945 A64 A65 L947 L948 L950 A70 L968 bodies 1 in component "PCB"
extrude "Extrude15" add sketch "dxf" along normal blind 4.5 contours A14 A20 A55 A63 | A15 A21 A56 A57 | A17 A24 A52 A62 | A18 A19 A54 A61 bodies 1 in component "PCB"
extrude "Extrude16" add sketch "dxf" along normal blind 6 contours L849 L895 L902 L904 L905 L908 L913 bodies 1 in component "PCB"
extrude "Extrude17" add sketch "dxf" along normal blind 3.5 contours L849 L892 L895 L905 bodies 1 in component "PCB"
extrude "Extrude18" add sketch "dxf" along normal blind 3.6 contours L857 L875 L878 L899 L900 L901 L909 L911 L912 L914 L970 L971 L973 L974 L977 L980 bodies 1 in component "PCB"
extrude "Extrude19" add sketch "PET_Diag_Clip" along normal blind 3.4 and the other way blind 4.1 contours L3 L303 L304 L305 L306 L310 | L307 L308 L309 L310 L311 L312 bodies 1 in component "PCB"
extrude "Extrude20" add sketch "PET_Diag_Clip" along normal blind 1.5 and the other way blind 2.2 contours L308 L313 L314 L315 L316 L317 L318 L319 L320 L321 L322 L323 L324 bodies 1 in component "PCB"
sketch "switch" plane through (0, 83.9, 0) normal (0, 1, 0) x (-1, 0, 0) in component "PCB"
  line L0 (-18.85, -2.2) -> (-23.85, -2.2)
  line L1 (-23.85, -2.2) -> (-23.85, 1.5)
  line L2 (-23.85, 1.5) -> (-18.85, 1.5)
  line L3 (-18.85, 1.5) -> (-18.85, -2.2)
  line L4 (-11.85, -4.1) -> (-11.85, 3.4)
  line L5 (-11.85, 3.4) -> (-35.15, 3.4)
  line L6 (-35.15, 3.4) -> (-35.15, -4.1)
  line L7 (-35.15, -4.1) -> (-11.85, -4.1)
  line L8 (-35.15, 3.4) -> (-11.85, 3.4) construction
  line L9 (-35.15, -4.1) -> (-35.15, 3.4) construction
  line L10 (-11.85, -4.1) -> (-35.15, -4.1) construction
  line L11 (-11.85, -4.1) -> (-11.85, 3.4) construction
  line L12 (-18.85, -2.2) -> (-18.85, 1.5) construction
  line L13 (-23.85, -2.2) -> (-23.85, 1.5) construction
  line L14 (-23.85, 1.5) -> (-18.85, 1.5) construction
  line L15 (-23.85, -2.2) -> (-18.85, -2.2) construction
  line L16 (-35.15, -0.35) -> (-11.85, -0.35) construction
  line L17 (-28.2, 1.8) -> (-18.8, 1.8)
  line L18 (-18.8, 1.8) -> (-18.8, -2.5)
  line L19 (-18.8, -2.5) -> (-28.2, -2.5)
  line L20 (-28.2, -2.5) -> (-28.2, 1.8)
  line L21 (-23.5, 3.4) -> (-23.5, -4.1) construction
  dimension "d227" = 9.4
  dimension "d228" = 4.3
  constraint coincident L1.end L2.start
  constraint coincident L2.end L3.start
  constraint coincident L0.end L1.start
  constraint coincident L0.start L3.end
  constraint midpoint L9 L16.start
  constraint midpoint L11 L16.end
  constraint horizontal L19
  constraint midpoint L8 L21.start
  constraint midpoint L10 L21.end
  constraint symmetric L16 L17 L19
  constraint symmetric L18 L20 L21
  measures "d227" distance of L17.start L17.end
  measures "d228" distance of L17 L19
extrude "Extrude21" cut sketch "switch" against normal blind 1 contours L17 L18 L19 L20 bodies 1 in component "PCB"
ref_plane "WorkPlane1" through (23.5, 38.5, -4.6) normal (0, 0, 1) x (1, 0, 0) in component "bottom_shell"